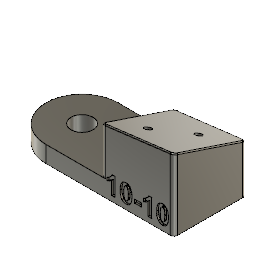
Angled Mirror Mount - Parametric (Autodesk Fusion 360 design; units mm, degrees)
Autodesk Fusion 360 part; units mm, degrees
sketch "Sketch1" plane through (0, 0, 0) normal (0, 0, 1) x (1, 0, 0)
  circle A0 centre (0, 0) radius 3.025
  line L0 (10, -10) -> (-10, -10)
  line L1 (-10, -10) -> (-10, 10)
  line L2 (-10, 10) -> (10, 10)
  line L3 (10, 10) -> (10, -10)
  line L4 (10, -10) -> (-10, 10) construction
  line L5 (-10, -10) -> (10, 10) construction
  line L6 (10, -10) -> (10, 10)
  line L7 (-10, 10) -> (-25.4, 10)
  line L8 (-25.4, -10) -> (-10, -10)
  line L9 (-10, -10) -> (-10, 10)
  line L10 (0, 0) -> (-25.4, 0) construction
  circle A1 centre (-25.4, 0) radius 3.025
  arc A2 (-25.4, 10) -> (-25.4, -10) centre (-25.4, 0) ccw
  dimension "d99" = 6.05
  dimension "d115" = 20
  dimension "d116" = 20
  dimension "d199" = 25.4
  dimension "d200" = 6.05
  constraint coincident A0.centre L10.start
  constraint horizontal L0
  constraint perpendicular L0 L1
  constraint parallel L0 L2
  constraint parallel L1 L3
  constraint coincident L4 A0.centre
  constraint coincident L5 A0.centre
  constraint vertical L6
  constraint horizontal L7
  constraint horizontal L8
  constraint vertical L9
  constraint horizontal L10
  constraint coincident L10.end A1.centre
  measures "d99" diameter of A0
  measures "d115" distance of L1.end L2.end
  measures "d116" distance of L0.end L1.end
  measures "d199" distance of A0.centre L10.end
  measures "d200" diameter of A1
extrude "Extrude3" add sketch "Sketch1" along normal blind 20 contours A0 | L0 L1 L2 L3 L6 L9 makes body 1
extrude "Extrude25" add sketch "Sketch1" along normal blind 4.625 contours L1 L7 L8 L9 A2 bodies 1
extrude "Extrude17" cut sketch "Sketch1" along normal blind 6 contours A0 bodies 1
sketch "Sketch11" plane through (10, 0, 0) normal (1, 0, 0) x (0, 1, 0)
  line L0 (10, 0) -> (10, 20)
  line L1 (10, 20) -> (-10, 20)
  line L2 (-10, 20) -> (-10, 0)
  line L3 (10, 20) -> (10, 13.3013)
  line L4 (-10, 20) -> (-10, 19.9999)
  line L5 (-10, 0) -> (10, 0)
  dimension "d121" = 6.6987
  dimension "d122" = 0.0001
  constraint vertical L3
  constraint coincident L0.end L1.start
  constraint coincident L1.end L2.start
  constraint perpendicular L1 L4
  measures "d121" distance of L0.end L3.end
  measures "d122" distance of L1.end L4.end
sketch "Sketch12" plane through (-10, 0, 0) normal (-1, 0, 0) x (0, -1, 0)
  line L0 (10, 4.625) -> (10, 20)
  line L1 (10, 20) -> (-10, 20)
  line L2 (-10, 20) -> (-10, 4.625)
  line L3 (10, 20) -> (10, 17.5085)
  line L4 (-10, 20) -> (-10, 10.8099)
  line L5 (-10, 4.625) -> (10, 4.625)
  dimension "d123" = 2.4915
  dimension "d124" = 9.1901
  constraint coincident L0.end L1.start
  constraint perpendicular L1 L3
  constraint coincident L1.end L2.start
  constraint perpendicular L1 L4
  measures "d123" distance of L0.end L3.end
  measures "d124" distance of L1.end L4.end
ref_plane "WorkPlane2" through (10, 10, 13.3013) normal (0.117303, -0.315399, -0.941681) x (0.937275, 0.348592, 0)
split "Split2" by plane through (10, 10, 13.3013) normal (0.117303, -0.315399, -0.941681) bodies 1 makes body 2 at (-11.8, -3.3333, 0)
sketch "Row-Column Text" plane through (0, -10, 0) normal (0, -1, 0) x (1, 0, 0)
  line L0 (-10, 17.5085) -> (-10, 4.625)
  line L1 (-25.4, 0) -> (10, 0)
  line L2 (10, 0) -> (10, 19.9999)
  line L3 (-5.2209, 0.9544) -> (5.2251, 0.9615) construction
  line L4 (5.2251, 0.9615) -> (5.2209, 7.0456) construction
  line L5 (5.2209, 7.0456) -> (-5.2251, 7.0385) construction
  line L6 (-5.2251, 7.0385) -> (-5.2209, 0.9544) construction
  line L7 (10, 19.9999) -> (-10, 17.5085)
  line L8 (-10, 4.625) -> (-25.4, 4.625)
  line L9 (-25.4, 4.625) -> (-25.4, 0)
  dimension "d130" = 5
  text T0 "10-10" font "Arial" height 5 bold align centre middle in box 10.446 x 6.0841 at (-5.2209, 0.9544) x (1, 0.000683) y (-0.000683, 1) spacing 1 kerned
extrude "Extrude19" cut sketch "Row-Column Text" against normal blind 0.5 text T0 bodies 2
ref_plane "WorkPlane3" through (0, 0, 12.125) normal (-0.707107, 0.707107, 0) x (0, 0, 1)
sketch "Sketch20" plane through (0, 0, 12.125) normal (-0.707107, 0.707107, 0) x (0, 0, 1)
  line L0 (5.3835, -14.1421) -> (1.2306, 13.89)
  point P0 (5.3835, -14.1421)
  point P1 (1.1763, 14.1421)
  constraint coincident P0 L0.start
sketch "Sketch21" plane through (-1.7017, 4.5753, 13.6605) normal (-0.117303, 0.315399, 0.941681) x (-0.937275, -0.348592, 0)
  line L0 (-5.8868, 18.8389) -> (-12.8587, -1.0676)
  line L1 (-12.8587, -1.0676) -> (5.8868, -8.4712)
  line L2 (5.8868, -8.4712) -> (12.8587, 11.4352)
  line L3 (12.8587, 11.4352) -> (-5.8868, 18.8389)
  line L4 (-12.6294, -0.9504) -> (12.8587, 11.4352)
  line L5 (0.1146, 5.2424) -> (4.6118, 7.4278)
  line L6 (0.1146, 5.2424) -> (-4.3825, 3.0571)
  circle A0 centre (4.6118, 7.4278) radius 0.925
  circle A1 centre (-4.3825, 3.0571) radius 0.925
  dimension "d167" = 5
  dimension "d168" = 5
  dimension "d169" = 1.85
  dimension "d170" = 1.85
  constraint midpoint L4 L5.start
  constraint parallel L4 L5
  constraint parallel L4 L6
  constraint coincident L5.end A0.centre
  constraint coincident L6.end A1.centre
  measures "d167" distance of L5.start L5.end
  measures "d168" distance of L5.start L6.end
  measures "d169" diameter of A0
  measures "d170" diameter of A1
extrude "Extrude22" cut sketch "Sketch21" against normal blind 6 contours L4 L6 A1 | L4 L6 A1 | L4 L5 A0 | L4 L5 A0 bodies 2
fillet "Fillet32" radius 1 4 edges at (-10, -10, 11.0668) (10, -10, 10) (-10, 10, 7.7175) (10, 10, 6.6506) on bodies 2
fillet "Fillet33" radius 0.25 8 edges at (-10, 0, 14.1592) (-9.7071, 9.7071, 10.9445) (0, 10, 12.0556) (9.7071, 9.7071, 13.3629) (10, 0, 16.6506) (9.7071, -9.7071, 19.8653) (0, -10, 18.7542) (-9.7071, -9.7071, 17.4469) on bodies 2
hidden bodies 1
equation "d99 = 0.25 in - 0.3 mm"
equation "Corner1 = 6.698626006910353 mm" comment "Import from spreadsheet/Python code"
equation "Corner2 = 0.0 mm" comment "Import from spreadsheet/Python code"
equation "Corner3 = 2.4913591178929444 mm" comment "Import from spreadsheet/Python code"
equation "Corner4 = 9.189985124803297 mm" comment "Import from spreadsheet/Python code"
equation "d121 = Corner1 + 0.0001 mm"
equation "d122 = Corner2 + 0.0001 mm"
equation "d123 = Corner3 + 0.0001 mm"
equation "d124 = Corner4 + 0.0001 mm"
named bodies: "Cut Off Angle", "Body"
